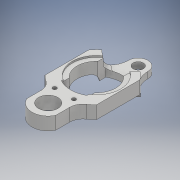
# Autodesk Inventor part: bottom_connect
Saved by Autodesk Inventor 2017 (Build 210142000, 142)
## iProperties
Created: 2018-05-30
Part Number: bottom_connect
Material: Generic
Document SubType Name: Modeling
Designer: Nic
Density: 1 g/cm^3
Appearance: Default
Author: Nic
Autodesk Inventor part; units mm, degrees
ref_plane "YZ Plane" through (0, 0, 0) normal (1, 0, 0) x (0, 1, 0)
ref_plane "XZ Plane" through (0, 0, 0) normal (0, 1, 0) x (-1, 0, 0)
ref_plane "XY Plane" through (0, 0, 0) normal (0, 0, 1) x (1, 0, 0)
sketch "Sketch1" plane through (0, 0, 0) normal (0, 0, 1) x (1, 0, 0)
  circle A0 centre (0, 0) radius 7.5 construction
  line L0 (8, 7) -> (8, -8)
  line L1 (-8, -8) -> (-8, 7)
  line L2 (0, 0) -> (0, 10.687) construction
  line L3 (0, 0) -> (8, 0) construction
  line L4 (-4, 6.9282) -> (-4, 4.4721)
  line L5 (4, 6.9282) -> (4, 4.4721)
  line L6 (-4, -6.9282) -> (-4, -4.4721)
  line L7 (4, -6.9282) -> (4, -4.4721)
  arc A1 (-4, 4.4721) -> (-4, -4.4721) centre (0, 0) ccw
  arc A2 (4, -4.4721) -> (4, 4.4721) centre (0, 0) ccw
  circle A3 centre (0, -15) radius 3
  arc A4 (-4, -6.9282) -> (4, -6.9282) centre (0, 0) ccw
  arc A5 (-4.5, -17.1794) -> (4.5, -17.1794) centre (0, -15) ccw
  line L8 (-4.5, -10.3803) -> (-4.5, -17.1794)
  line L9 (4.5, -10.3803) -> (4.5, -17.1794)
  arc A6 (-8, -8) -> (-4.5, -10.3803) centre (0, 0) ccw
  arc A7 (4.5, -10.3803) -> (8, -8) centre (0, 0) ccw
  circle A8 centre (0, 13) radius 1.6
  arc A9 (4, 6.9282) -> (-4, 6.9282) centre (0, 0) ccw
  arc A10 (2.9999, 12.972) -> (-2.9999, 12.972) centre (0, 13) ccw
  arc A11 (-8, 7) -> (-2.9999, 12.972) centre (-8.9996, 12.9161) ccw
  arc A12 (2.9999, 12.972) -> (8, 7) centre (8.9996, 12.9161) ccw
  arc A13 (-6.947, 7.2782) -> (-4, 4.9377) centre (0, 13) ccw
  arc A14 (4, 4.9377) -> (6.947, 7.2782) centre (0, 13) ccw
  dimension "d0" = 15
  dimension "d1" = 16
  dimension "d2" = 15
  dimension "d3" = 8
  dimension "d4" = 6
  dimension "d5" = 6
  dimension "d6" = 16
  dimension "d8" = 15
  dimension "d9" = 10
  dimension "d10" = 9
  dimension "d11" = 13
  dimension "d12" = 3.2
  dimension "d13" = 6
  dimension "d15" = 11.3137
  dimension "d16" = 8
  dimension "d17" = 6
  dimension "d42" = 9
  constraints: 26 point on circle, 21 end point, 15 centre point, 8 coincident, 8 symmetric about line, 5 point on line, 3 vertical, 2 concentric, 2 parallel, 1 horizontal, 1 tangent, 1 vertical alignment, 4 other
  measures "d0" diameter of A0
  measures "d1" distance of L1.start L0.end
  measures "d2" distance of L1.start L1.end
  measures "d3" distance between parallel lines of L5 L4
  measures "d4" radius of A2
  measures "d5" diameter of A3
  measures "d6" distance between parallel lines of L0 L1
  measures "d8" distance of point (0, 0) A3.centre
  measures "d9" diameter of A5
  measures "d10" distance between parallel lines of L9 L8
  measures "d11" distance of point (0, 0) A8.centre
  measures "d12" diameter of A8
  measures "d13" diameter of A10
  measures "d15" radius of A7
  measures "d16" radius of A4
  measures "d17" radius of A11
  measures "d42" radius of A13
extrude "Extrusion1" add sketch "Sketch1" along normal blind 4 contours L0 A7 L9 A5 L8 A6 L1 A11 A13 L4 A1 L6 A4 L7 A2 L5 A14 A12 | A14 L5 A9 L4 A13 A11 A10 A12
extrude "Extrusion2" add sketch "Sketch1" against normal blind 2 contours A14 L5 A9 L4 A13 A11 A10 A12
sketch "Sketch2" plane through (0, 0, 4) normal (0, 0, 1) x (1, 0, 0)
  line L0 (8, 13) -> (8, 28)
  line L1 (8, 28) -> (-8, 28)
  line L2 (-8, 28) -> (-8, 13)
  arc A0 (-8, 13) -> (8, 13) centre (0, 13) ccw
  circle A1 centre (0, 13) radius 1.6 projected
  point P0 (0, 0)
  dimension "d25" = 15
  dimension "d40" = 8
  constraints: 6 end point, 2 point on circle, 2 tangent, 1 centre point, 1 concentric, 1 horizontal, 1 parallel, 1 vertical
  measures "d25" distance of L1.end L2.end
  measures "d40" radius of A0
extrude "Extrusion3" cut sketch "Sketch2" against normal blind 4 contours A0 L2 L1 L0 | A1
fillet "Fillet1" radius 2 4 edges at (5.0704, 6.812, 0) (-5.0704, 6.812, 0) (5.5972, 5.9522, 0) (-5.5972, 5.9522, 0)
fillet "Fillet2" radius 4 2 edges at (4.5, -10.3803, 2) (-4.5, -10.3803, 2)
sketch "Sketch3" plane through (0, 0, 4) normal (0, 0, 1) x (1, 0, 0)
  circle A0 centre (3, -10) radius 0.6
  point P0 (0, 0)
  dimension "d32" = 1.2
  dimension "d33" = 10
  dimension "d34" = 3
  constraints: 1 centre point
  measures "d32" diameter of A0
  measures "d33" vertical distance of point (0, 0) A0.centre
  measures "d34" horizontal distance of point (0, 0) A0.centre
extrude "Extrusion4" cut sketch "Sketch3" against normal up to next
mirror "Mirror1" about plane through (0, 0, 0) normal (1, 0, 0) of "Extrusion4"
sketch "Sketch4" plane through (0, 0, 4) normal (0, 0, 1) x (1, 0, 0)
  circle A0 centre (0, 0) radius 7.5
  dimension "d37" = 15
  constraints: 1 centre point, 1 coincident
  measures "d37" diameter of A0
extrude "Extrusion5" cut sketch "Sketch4" against normal blind 0.5
sketch "Sketch5" plane through (0, 0, 4) normal (0, 0, 1) x (1, 0, 0)
  line L0 (-9.7218, 0) -> (-15.5, 0)
  line L1 (-15.5, 0) -> (-15.5, 12)
  line L2 (-15.5, 12) -> (-5.5, 12)
  line L3 (-5.5, 12) -> (-5.5, 8.0164)
  line L4 (0, 0) -> (0, 13.5291) construction
  line L5 (9.7218, 0) -> (15.5, 0)
  line L6 (15.5, 0) -> (15.5, 12)
  line L7 (15.5, 12) -> (5.5, 12)
  arc A0 (2.9999, 12.972) -> (4.4628, 8.9896) centre (8.9996, 12.9161) ccw projected
  line L8 (5.5, 12) -> (5.5, 8.0164)
  line L9 (15.5, 0) -> (9.9132, 0)
  arc A1 (9.7218, 0) -> (5.5, 8.0164) centre (0, 0) ccw
  arc A2 (-5.5, 8.0164) -> (-9.7218, 0) centre (0, 0) ccw
  point P0 (-9.9132, 0)
  point P1 (4.6793, 8.7445)
  dimension "d45" = 10
  dimension "d46" = 12
  dimension "d50" = 11
  dimension "d51" = 9.7218
  constraints: 20 end point, 4 point on circle, 4 symmetric about line, 3 vertical, 2 centre point, 2 coincident, 2 horizontal, 2 perpendicular, 2 point on line, 1 concentric, 1 horizontal alignment, 1 other
  measures "d45" distance of L6.end L7.end
  measures "d46" distance between parallel lines of L0 L2
  measures "d50" distance between parallel lines of L3 L8
  measures "d51" radius of A1
extrude "Extrusion6" cut sketch "Sketch5" against normal through all
body "Solid1"
